Autodesk Inventor part; units mm, degrees
(part 2 of 2)
  arc A233 (-6.897, 40.5524) -> (-6.2461, 41.8236) centre (-11.877, 43.9045) ccw construction
  arc A234 (-6.2461, 41.8236) -> (-6.6124, 42.1677) centre (-13, 35.0012) ccw construction
  arc A235 (-6.6124, 42.1677) -> (-7.8405, 41.4388) centre (-4.1842, 36.6777) ccw construction
  arc A236 (-7.8405, 41.4388) -> (-8.1845, 41.7) centre (-13, 35.0012) ccw construction
  arc A237 (-8.1845, 41.7) -> (-7.8122, 43.0787) centre (-13.7526, 43.9434) ccw construction
  arc A238 (-7.8122, 43.0787) -> (-8.242, 43.3392) centre (-13, 35.0012) ccw construction
  arc A239 (-8.242, 43.3392) -> (-9.2917, 42.3708) centre (-4.7254, 38.474) ccw construction
  arc A240 (-9.2917, 42.3708) -> (-9.6825, 42.5548) centre (-13, 35.0012) ccw construction
  circle A241 centre (-13, 35.0012) radius 5 projected
  circle A242 centre (-14.5, 55.2958) radius 14.5 projected
  circle A243 centre (-14.5, 55.2958) radius 13.85 projected
  circle A244 centre (-14.5, 14.5) radius 14.5 projected
  circle A245 centre (-14.5, 14.5) radius 13.85 projected
  circle A246 centre (-14.5, 14.5) radius 5 projected
  line L0 (0, 0) -> (-23.2, 0) projected
  line L1 (0, 0) -> (-23.2, 0)
  line L2 (-23.2, 0) -> (-23.2, 65.2958)
  line L3 (-23.2, 65.2958) -> (0, 65.2958)
  line L4 (0, 65.2958) -> (0, 0)
  circle A247 centre (-9.2084, 22.9852) radius 8 construction
  circle A248 centre (-13, 35.0012) radius 9.6 construction
  circle A249 centre (-9.2084, 22.9852) radius 8.4
  circle A250 centre (-13, 35.0012) radius 10
  point P0 (23.5865, 13.8726)
  point P1 (-23.2, 26.1)
  point P2 (-20.0405, 27.8997)
  point P3 (-4.4107, 29.8803)
  point P4 (-9.5008, 14.5903)
  point P5 (-16.6184, 19.029)
  point P6 (-17.0946, 25.8779)
  point P7 (-19.5113, 27.4116)
  point P8 (-23.2, 25.2765)
  point P9 (-23.2, 0)
  point P10 (-1.2325, 20.35)
  point P11 (0, 14.5)
  point P12 (-15.7161, 28.2965)
  point P13 (-15.0841, 28.9882)
  point P14 (-7.0681, 26.9506)
  point P15 (-7.6627, 26.5447)
  point P16 (-1.5756, 19.4781)
  point P17 (-23.2, 3.7235)
  point P18 (-23.2, 2.9)
  point P19 (-14.5, 0)
  dimension "d14" = 0.4
  dimension "d15" = 0.4
  dimension "d16" = 0.2
  dimension "d17" = 4.5
  constraints: 8 end point, 2 centre point, 2 coincident, 2 parallel, 1 horizontal, 1 perpendicular, 7 other
  measures "d16" distance edge to line of A250 L2
  measures "d17" distance edge to line of A242 L3
extrude "Extrusion5" add sketch "Sketch2" along normal blind 4.5 contours A250 A242 L4 A244 A249 | A250 A245 L2 A244 | A244 L2 A242 A250 | A244 L2 A245 A249 | A242 L2 A243 A250 | A250 A249 A246 A245 L2 | A250 A243 L3 A242 | L4 L0 A244 | A244 L0 L2 | A243 L2 L3 A250 | A242 L3 L4
sketch "Sketch3" plane through (-23.5865, -7.0714, 13.8726) normal (0, 1, 0) x (1, 0, 0)
  line L0 (-1.5, 16.5) -> (-1.5, 0.5) projected
  line L1 (-2.5, 16.5) -> (-1.5, 16.5) projected
  line L2 (-2.5, 0.5) -> (-2.5, 16.5) projected
  line L3 (-2.5, 0.5) -> (-1.5, 0.5) projected
  line L4 (-1.5, 0.5) -> (-1, 0.5)
  line L5 (-1, 0.5) -> (-1, 17)
  line L6 (-1, 17) -> (-2.5, 17)
  line L7 (-2.5, 17) -> (-2.5, 16.5)
  point P0 (23.5865, 13.8726)
  dimension "d20" = 0.5
  dimension "d21" = 0.5
  constraints: 8 end point, 3 perpendicular, 1 horizontal
  measures "d20" distance between parallel lines of L6 L1
  measures "d21" distance between parallel lines of L5 L0
extrude "Extrusion6" cut sketch "Sketch3" against normal blind 7.5
sketch "Sketch4" plane through (-23.5865, -7.0714, 13.8726) normal (0, 1, 0) x (1, 0, 0)
  line L0 (-1.5, 16.5) -> (-1.5, 0.5) projected
  line L1 (-2.5, 16.5) -> (-1.5, 16.5) projected
  line L2 (-2.5, 0.5) -> (-2.5, 16.5) projected
  line L3 (-2.5, 0.5) -> (-1.5, 0.5) projected
  line L4 (-1.5, 3.6) -> (-1.5, 7.1) projected
  line L5 (-1.5, 3.6) -> (0, 3.6) projected
  line L6 (0, 7.1) -> (0, 3.6) projected
  line L7 (-1.5, 7.1) -> (0, 7.1) projected
  line L8 (-1.5, 9.9) -> (-1.5, 13.4) projected
  line L9 (-1.5, 9.9) -> (0, 9.9) projected
  line L10 (0, 13.4) -> (0, 9.9) projected
  line L11 (-1.5, 13.4) -> (0, 13.4) projected
  line L12 (0.5, 3.1) -> (-2, 3.1)
  line L13 (-2, 3.1) -> (-2, 7.6)
  line L14 (-2, 7.6) -> (0.5, 7.6)
  line L15 (0.5, 7.6) -> (0.5, 3.1)
  line L16 (0.5, 9.4) -> (-2, 9.4)
  line L17 (-2, 9.4) -> (-2, 13.9)
  line L18 (-2, 13.9) -> (0.5, 13.9)
  line L19 (0.5, 13.9) -> (0.5, 9.4)
  line L20 (-1, 0.5) -> (-2.5, 0.5) projected
  line L21 (-1.5, 0.5) -> (-1, 0.5)
  line L22 (-1, 0.5) -> (-1, 17)
  line L23 (-1, 17) -> (-2.5, 17)
  line L24 (-2.5, 17) -> (-2.5, 16.5)
  line L25 (-2.5, 0.5) -> (-2.5, 0)
  line L26 (0, 0) -> (-23.2, 0) projected
  line L27 (-2.5, 0) -> (0, 0)
  line L28 (0, 0) -> (0, 16.9971)
  line L29 (0, 65.2958) -> (0, 0) projected
  line L30 (-2.5, 17) -> (-2.5, 17.9298)
  line L31 (-2.4477, 18) -> (0, 18)
  arc A0 (-9.5008, 14.5903) -> (-4.4107, 29.8803) centre (-9.2084, 22.9852) ccw projected
  point P0 (23.5865, 13.8726)
  point P1 (0, 3.1)
  point P2 (-1, 3.1)
  point P3 (0, 7.6)
  point P4 (0, 9.4)
  point P5 (-1, 9.4)
  point P6 (-1, 7.6)
  point P7 (-1, 13.9)
  point P8 (0, 13.9)
  point P9 (-15.0841, 28.9882)
  point P10 (-1.5756, 19.4781)
  dimension "d24" = 0.5
  dimension "d25" = 0.5
  dimension "d26" = 0.5
  dimension "d27" = 1
  constraints: 34 end point, 4 perpendicular, 3 point on line, 2 vertical, 1 collinear, 1 horizontal, 1 point on circle, 6 other
  measures "d24" distance between parallel lines of L5 L12
  measures "d25" distance between parallel lines of L9 L16
  measures "d26" distance between parallel lines of L1 L23
  measures "d27" distance between parallel lines of L23 L31
extrude "Extrusion7" add sketch "Sketch4" along normal blind 8 contours L22 L23 L30 A0 L31 L29 L28 L18 | L16 L28 L14 L22 | L3 L20 L22 L12 L28 L26 L25
sketch "Sketch6" plane through (-23.5865, -7.0714, 13.8726) normal (0, 1, 0) x (1, 0, 0)
  circle A0 centre (-20.6284, 19.6423) radius 2.25 projected
  circle A1 centre (-8.3716, 9.3577) radius 2.25 projected
  point P0 (23.5865, 13.8726)
extrude "Extrusion8" cut sketch "Sketch6" against normal blind 2.6
sketch "Sketch7" plane through (-44.2149, -9.6714, -5.7697) normal (0, 1, 0) x (1, 0, 0)
  circle A0 centre (0, 0) radius 2.25 projected
  circle A1 centre (12.2567, -10.2846) radius 2.25 projected
  point P0 (44.2149, -5.7697)
hole "Hole2" at (-44.2149, -9.6714, -5.7697) at (-31.9582, -9.6714, 4.5149) direction (0, -1, 0) diameter 2.5 depth 10.6 counterbore diameter 4.5 counterbore depth 2.6
sketch "Sketch5" plane through (-23.5865, -16.1714, -51.4232) normal (0, 0, -1) x (-1, 0, 0)
  line L0 (4.9176, 0) -> (0, 0) projected
  line L1 (23.2, 0.6) -> (23.2, 9.1) projected
  line L2 (0, 9.1) -> (23.2, 9.1) projected
  line L3 (23.2, 4.6) -> (6.7249, 4.6) projected
  line L4 (6, 9.1) -> (6, 0.6)
  circle A0 centre (16.7, 6.85) radius 3.5
  circle A1 centre (9.5, 6.85) radius 3.5
  line L5 (23.2, 0.6) -> (23.2, 9.1) projected
  line L6 (0, 0) -> (0, 9.1) projected
  line L7 (4.9176, 0.6) -> (4.9176, 0) projected
  line L8 (4.9176, 0.6) -> (23.2, 0.6) projected
  point P0 (-23.5865, 16.1714)
  point P1 (5.9014, 4.6)
  dimension "d49" = 7
  dimension "d50" = 7
  dimension "d51" = 2.25
  dimension "d52" = 2.25
  dimension "d53" = 2.25
  dimension "d54" = 2.25
  dimension "d55" = 3
  dimension "d67" = 6
  constraints: 2 centre point, 2 end point, 1 point on line, 1 tangent
  measures "d49" diameter of A0
  measures "d50" diameter of A1
  measures "d51" distance from line of L3 A1.centre
  measures "d52" distance from line of L2 A1.centre
  measures "d53" distance from line of A0.centre L3
  measures "d54" distance from line of L2 A0.centre
  measures "d55" distance edge to line of A0 L1
  measures "d67" distance between parallel lines of L6 L4
hole "Hole1" at (-40.2865, -9.3214, -51.4232) at (-33.0865, -9.3214, -51.4232) direction (0, 0, 1) diameter 4 depth 5.5 counterbore diameter 4.5 counterbore depth 0.5
sketch "Sketch9" plane through (-23.5865, -14.4714, 13.8726) normal (0, 1, 0) x (1, 0, 0)
  arc A0 (-2.4477, 18) -> (-4.4107, 29.8803) centre (-9.2084, 22.9852) ccw projected
  point P0 (23.5865, 13.8726)
  point P1 (-1.5756, 19.4781)
hole "Hole3" at (-32.7949, -14.4714, -9.1126) direction (0, -1, 0) diameter 2.5 depth 1.5
sketch "Sketch10" plane through (-23.5865, -7.0714, 13.8726) normal (0, 1, 0) x (1, 0, 0)
  circle A0 centre (-8.3716, 9.3577) radius 2.25 projected
  circle A1 centre (-20.6284, 19.6423) radius 2.25 projected
  line L0 (-2.5, 0) -> (-2.5, 0.5) projected
  line L1 (-2.5, 0.5) -> (-2.5, 17) projected
  line L2 (-2.5, 17) -> (-2.5, 17.9298) projected
  arc A2 (-9.5008, 14.5903) -> (-2.5, 17.9298) centre (-9.2084, 22.9852) ccw projected
  arc A3 (-16.6184, 19.029) -> (-9.5008, 14.5903) centre (-14.5, 14.5) ccw projected
  arc A4 (-17.0946, 25.8779) -> (-16.6184, 19.029) centre (-9.2084, 22.9852) ccw projected
  arc A5 (-4.4107, 29.8803) -> (-17.0946, 25.8779) centre (-13, 35.0012) ccw projected
  arc A6 (-2.4477, 18) -> (-4.4107, 29.8803) centre (-9.2084, 22.9852) ccw projected
  line L3 (-2.4477, 18) -> (0, 18) projected
  line L4 (0, 18) -> (0, 65.2958) projected
  line L5 (0, 65.2958) -> (-9.5, 65.2958) projected
  line L6 (-9.5, 64.7958) -> (-9.5, 65.2958) projected
  line L7 (-9.5, 65.2958) -> (-16.7, 65.2958) projected
  line L8 (-16.7, 64.7958) -> (-16.7, 65.2958) projected
  line L9 (-16.7, 65.2958) -> (-23.2, 65.2958) projected
  line L10 (-23.2, 65.2958) -> (-23.2, 0) projected
  line L11 (-23.2, 0) -> (-2.5, 0) projected
  circle A7 centre (-3.5, 61.7958) radius 3.5
  line L12 (0, 18) -> (0, 65.2958) projected
  circle A8 centre (-19.2, 8.25) radius 3.5
  circle A9 centre (-19.7, 46.7213) radius 3.5
  circle A10 centre (-3.5, 44.5929) radius 3.5
  circle A11 centre (-14.5, 55.2958) radius 3.5
  circle A12 centre (-14.5, 55.2958) radius 5 construction
  line L13 (-23.2, 4.75) -> (-2.5, 4.75)
  line L14 (-2.5, 13) -> (-23.2, 13)
  circle A13 centre (-19.2, 8.25) radius 2.5
  point P0 (23.5865, 13.8726)
  point P1 (-8.7001, 9.5502)
  dimension "d75" = 7
  dimension "d76" = 7
  dimension "d78" = 7
  dimension "d79" = 7
  dimension "d80" = 7
  dimension "d88" = 4.75
  dimension "d89" = 8.25
  dimension "d90" = 3.5
  dimension "d91" = 4.75
  dimension "d93" = 4
  dimension "d96" = 5
  constraints: 6 centre point, 6 tangent, 4 end point, 4 point on line, 2 coincident, 2 perpendicular
  measures "d75" diameter of A7
  measures "d76" diameter of A8
  measures "d78" diameter of A9
  measures "d79" diameter of A10
  measures "d80" diameter of A11
  measures "d88" distance between parallel lines of L11 L13
  measures "d89" distance between parallel lines of L14 L13
  measures "d90" distance from line of L13 A8.centre
  measures "d91" distance from line of L14 A8.centre
  measures "d93" distance from line of L10 A8.centre
  measures "d96" diameter of A13
hole "Hole4" at (-43.2865, -7.0714, -32.8486) at (-27.0865, -7.0714, -47.9232) at (-38.0865, -7.0714, -41.4232) at (-27.0865, -7.0714, -30.7202) at (-32.2867, -7.0714, 4.3225) at (-42.7865, -7.0714, 5.6226) direction (0, -1, 0) diameter 4 depth 3.5 counterbore diameter 4.5 counterbore depth 0.5
equation "\"d51\" = d52"
equation "\"d53\" = d54"
body "Solid2"
